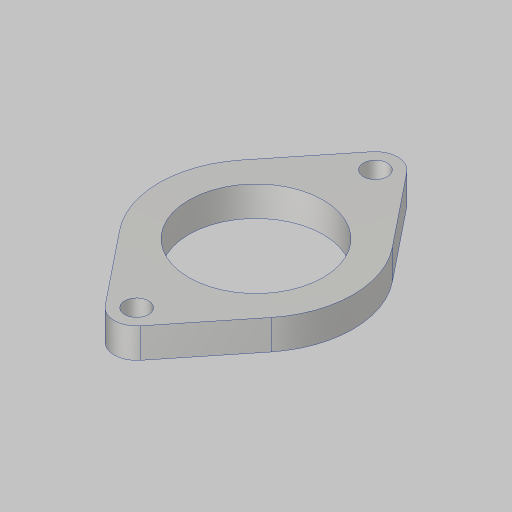
# Autodesk Inventor part: EL2-CGB-005
Saved by Autodesk Inventor 2023.5 (Build 275446000, 446)
## iProperties
Created: 2025-01-23
Part Number: EL2-CGB-005
Material: Aluminum 6061
Document SubType Name: Modeling
Designer: slick
Density: 2.7 g/cm^3
Appearance: Aluminum - Flat
Author: slick
Autodesk Inventor part; units mm, degrees
ref_plane "YZ Plane" through (0, 0, 0) normal (1, 0, 0) x (0, 1, 0)
ref_plane "XZ Plane" through (0, 0, 0) normal (0, 1, 0) x (-1, 0, 0)
ref_plane "XY Plane" through (0, 0, 0) normal (0, 0, 1) x (1, 0, 0)
sketch "Sketch1" plane through (0, 0, 0) normal (0, 1, 0) x (-1, 0, 0)
  circle A0 centre (0, 0) radius 14.2875
  line L0 (0, 25.4) -> (0, -25.4) construction
  circle A1 centre (0, 0) radius 18.1864 construction
  circle A2 centre (0, 25.4) radius 4.7625 construction
  circle A3 centre (0, -25.4) radius 4.7625 construction
  circle A4 centre (0, 0) radius 20.6375 construction
  line L1 (16.1101, 12.8984) -> (3.7177, 28.3766)
  line L2 (16.1101, -12.8984) -> (3.7177, -28.3766)
  line L3 (-3.7177, -28.3766) -> (-16.1101, -12.8984)
  line L4 (-16.1101, 12.8984) -> (-3.7177, 28.3766)
  arc A5 (3.7177, 28.3766) -> (-3.7177, 28.3766) centre (0, 25.4) ccw
  arc A6 (-16.1101, 12.8984) -> (-16.1101, -12.8984) centre (0, 0) ccw
  arc A7 (16.1101, -12.8984) -> (16.1101, 12.8984) centre (0, 0) ccw
  arc A8 (-3.7177, -28.3766) -> (3.7177, -28.3766) centre (0, -25.4) ccw
  point P0 (-3.7177, 28.3766)
  point P1 (3.7177, -28.3766)
  dimension "d0" = 28.575
  dimension "d1" = 50.8
  dimension "d2" = 36.3728
  dimension "d3" = 9.525
  dimension "d4" = 9.525
  dimension "d5" = 6.35
  constraints: 20 point on circle, 10 end point, 9 centre point, 8 coincident, 8 tangent, 2 concentric, 2 midpoint, 1 point on line, 1 vertical
  measures "d0" diameter of A0
  measures "d1" distance of L0.start L0.end
  measures "d2" diameter of A1
  measures "d3" diameter of A2
  measures "d4" diameter of A3
  measures "d5" radial gap between concentric circles of A0 A4
extrude "Extrusion1" add sketch "Sketch1" along normal blind 6.35
hole "Hole1" at (0, 0, 25.4) at (0, 0, -25.4) direction (0, 1, 0) diameter 5.1054 end through all clearance for "Flat Head Machine Screw (82)" size "#10" standard "Ansi Unified Screw Threads"
body "Solid1"
